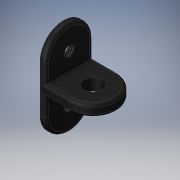
# Autodesk Inventor part: Door Hinge
Saved by Autodesk Inventor 2018 (Build 220112000, 112)
## iProperties
Created: 2018-02-09
Part Number: Door Hinge
Material: Steel, Alloy
Document SubType Name: Modeling
Designer: Joey
Density: 7.73 g/cm^3
Appearance: Diamond plate - Dark Gray
Author: Joey
Autodesk Inventor part; units mm, degrees
ref_plane "YZ Plane" through (0, 0, 0) normal (1, 0, 0) x (0, 1, 0)
ref_plane "XZ Plane" through (0, 0, 0) normal (0, 1, 0) x (-1, 0, 0)
ref_plane "XY Plane" through (0, 0, 0) normal (0, 0, 1) x (1, 0, 0)
sketch "Sketch1" plane through (0, 0, 0) normal (0, 0, 1) x (1, 0, 0)
  line L0 (0, -50.8) -> (0, 50.8)
  line L1 (0, 50.8) -> (6.35, 50.8)
  line L2 (6.35, 50.8) -> (6.35, 6.35)
  line L3 (6.35, 6.35) -> (57.15, 6.35)
  line L4 (57.15, 6.35) -> (57.15, -6.35)
  line L5 (57.15, -6.35) -> (6.35, -6.35)
  line L6 (6.35, -6.35) -> (6.35, -50.8)
  line L7 (6.35, -50.8) -> (0, -50.8)
  line L8 (0, 0) -> (57.15, 0) construction
  dimension "d0" = 12.7
  dimension "d1" = 101.6
  dimension "d2" = 50.8
  dimension "d3" = 6.35
  constraints: 18 end point, 6 perpendicular, 2 midpoint, 2 point on line, 1 coincident, 1 horizontal, 1 vertical
  measures "d0" distance of L3.end L4.end
  measures "d1" distance of L0.start L0.end
  measures "d2" distance of L2.end L3.end
  measures "d3" distance of L0.end L1.end
extrude "Extrusion1" add sketch "Sketch1" along normal mid plane 50.8
fillet "Fillet1" radius 25.4 6 edges at (57.15, 0, 25.4) (57.15, 0, -25.4) (3.175, 50.8, -25.4) (3.175, 50.8, 25.4) (3.175, -50.8, 25.4) (3.175, -50.8, -25.4)
fillet "Fillet2" radius 3.175 12 edges at (49.7105, 6.35, 17.9605) (19.05, 6.35, -25.4) (19.05, 6.35, 25.4) (49.7105, -6.35, 17.9605) (19.05, -6.35, -25.4) (19.05, -6.35, 25.4) (6.35, 15.875, -25.4) (6.35, 15.875, 25.4) (6.35, 43.3605, -17.9605) (6.35, -15.875, 25.4) (6.35, -15.875, -25.4) (6.35, -43.3605, 17.9605)
hole "Hole1" at (31.75, 6.35, 0) direction (0, -1, 0) diameter 19.05 end through all
sketch "Sketch2" plane through (6.35, 6.35, 22.225) normal (1, 0, 0) x (0, 0, -1)
  line L0 (22.225, 19.05) -> (22.225, -31.75) construction
  point P0 (22.225, -6.35)
  point P1 (22.225, -6.35)
  dimension "d17" = 50.8
  constraints: 2 end point, 1 coincident, 1 midpoint, 1 vertical
  measures "d17" distance of L0.start L0.end
hole "Hole2" at (6.35, 25.4, 0) at (6.35, -25.4, 0) direction (-1, 0, 0) diameter 10.5918 end through all thread size "1/2-13 UNC" class "2B" standard "ANSI Unified Screw Threads"
body "Solid1"
